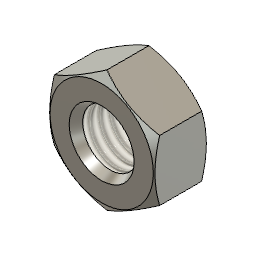
HalterungenSpritzenkopf (Autodesk Fusion 360 archive; units mm, degrees)
design "Sechskantmutter DIN 934 - M8 x 1.25 Stahl 6 Einfach"
description: Sechskantmutter DIN 934 - M8 x 1.25
part number: DIN 934 - M8 x 1.25 Stahl 6 Einfach
Autodesk Fusion 360 part; units mm, degrees
sketch "Sketch1" plane through (0, 0, 0) normal (0, 1, 0) x (1, 0, 0)
  line L0 (0, 0) -> (0, -6.5)
  line L1 (-4, 0) -> (-6.37, 0)
  line L2 (-6.37, 0) -> (-7.5075, -0.6567)
  line L3 (-7.5075, -0.6567) -> (-7.5075, -5.8433)
  line L4 (-7.5075, -5.8433) -> (-6.37, -6.5)
  line L5 (-6.37, -6.5) -> (-4, -6.5)
  line L6 (-4, -6.5) -> (-4, 0)
  dimension "d121" = 8
  dimension "d122" = 30
  dimension "d123" = 30
  dimension "d128" = 15.015
  dimension "d172" = 12.74
  dimension "d179" = 6.5
  constraint vertical L0
  constraint coincident L0 L0.end
  constraint coincident origin L0
  constraint horizontal L1
  constraint coincident L0.start L1
  constraint coincident L0.start origin
  constraint coincident L0.end L5
  constraint vertical L1.end L4.end
  measures "d122" angle of L1 L2
  measures "d123" angle of L4 L5
  measures "d179" distance of L1 L5
revolve "Revolve1" add sketch "Sketch1" angle 360 about axis through (0, 0, 0) along (0, 0, 1)
sketch "Sketch8" plane through (0, 0, 6.5) normal (0, 0, 1) x (1, 0, 0)
  line L0 (-6.5, -3.7567) -> (-6.5, 3.7567)
  circle A0 centre (0, 0) radius 4
  circle A1 centre (0, 0) radius 7.5075
  dimension "d114" = 6.5
  constraint coincident L0.end A1
  constraint coincident L0.start A1
  constraint vertical L0
  measures "d114" distance of A0.centre L0
extrude "Extrude5" cut sketch "Sketch8" against normal blind 6.5 contours L0 A1 picked at (-6.6626, -0.915)
pattern_circular "C-Pattern2" count 6 over 360 about axis through (0, 0, 1.75) along (0, 0, 1) of "Extrude5"
thread "Thread3" "ISO Metric profile 8.0 M8x1.25 M8x1.25 6H" major diameter 8.17 minor diameter 6.7795 pitch 1.25 angle 60 resizes the face on face at (-3.9801, 0.3983, 4.3333)
sketch "Sketch12" plane through (0, 0, 0) normal (0, 1, 0) x (1, 0, 0)
  line L0 (-4, 0) -> (0, 0)
  line L1 (-2.1236, -3.25) -> (-4, 0)
  line L2 (-4, -6.5) -> (0, -6.5)
  line L3 (-2.1236, -3.25) -> (-4, -6.5)
  line L4 (0, 0) -> (0, -6.5)
  dimension "d169" = 60
  dimension "d177" = 4
  dimension "d178" = 60
  constraint horizontal L0
  constraint coincident L1.start L3.start
  constraint vertical L0.start L2.start
  constraint coincident L2.end L4.end
  constraint coincident L0.end L4.start
  constraint perpendicular L2 L4
  measures "d169" angle of L2 L3
  measures "d177" distance of L0.start L4
  measures "d178" angle of L0 L1
revolve "Revolve3" cut sketch "Sketch12" angle 360 about axis through (0, 0, 1.75) along (0, 0, 1)
equation "adsk_nheig = 6.50 mm"
equation "adsk_maxdia = 15.015 mm"
equation "adsk_nomdia = 8.00 mm"
equation "d89 = -adsk_nheig"
equation "adsk_waflat = 13.00 mm"
equation "d114 = adsk_waflat / 2"
equation "adsk_chamang1 = 30.00 deg"
equation "adsk_chamang2 = 30.00 deg"
equation "d121 = adsk_nomdia"
equation "d122 = adsk_chamang1"
equation "d123 = adsk_chamang2"
equation "d128 = adsk_maxdia"
equation "d163 = adsk_nheig"
equation "adsk_beardia = adsk_waflat * 0.98"
equation "d172 = adsk_beardia"
equation "d177 = adsk_nomdia * 0.5"
equation "d179 = adsk_nheig"
